extractorororororor0r0r0r (Autodesk Fusion 360 design; units mm, degrees)
Autodesk Fusion 360 part; units mm, degrees
sketch "Sketch1" plane through (0, 0, 0) normal (0, 1, 0) x (1, 0, 0)
  circle A0 centre (0, 0) radius 63.5
  line L0 (63.5, 63.5) -> (-63.5, 63.5)
  line L1 (-63.5, 63.5) -> (-63.5, -63.5)
  line L2 (-63.5, -63.5) -> (63.5, -63.5)
  line L3 (63.5, -63.5) -> (63.5, 63.5)
  line L4 (63.5, 63.5) -> (-63.5, -63.5) construction
  line L5 (-63.5, 63.5) -> (63.5, -63.5) construction
  line L6 (70, 70) -> (-70, 70)
  line L7 (-70, 70) -> (-70, -70)
  line L8 (-70, -70) -> (70, -70)
  line L9 (70, -70) -> (70, 70)
  line L10 (70, 70) -> (-70, -70) construction
  line L11 (-70, 70) -> (70, -70) construction
  circle A1 centre (0, 0) radius 70
  line L12 (60, 60) -> (-60, 60)
  line L13 (-60, 60) -> (-60, -60)
  line L14 (-60, -60) -> (60, -60)
  line L15 (60, -60) -> (60, 60)
  line L16 (60, 60) -> (-60, -60) construction
  line L17 (-60, 60) -> (60, -60) construction
  dimension "d1" = 127
  dimension "d2" = 127
  dimension "d3" = 127
  dimension "d4" = 140
  dimension "d5" = 140
  dimension "d14" = 120
  dimension "d15" = 120
  constraint coincident A0.centre A1.centre
  constraint perpendicular L0 L1
  constraint parallel L0 L2
  constraint parallel L1 L3
  constraint horizontal L0
  constraint coincident L4 A0.centre
  constraint coincident L5 A0.centre
  constraint perpendicular L6 L7
  constraint parallel L6 L8
  constraint parallel L7 L9
  constraint horizontal L6
  constraint coincident L10 A0.centre
  constraint coincident L11 A0.centre
  constraint tangent L8 A1
  constraint perpendicular L12 L13
  constraint parallel L12 L14
  constraint parallel L13 L15
  constraint horizontal L12
  constraint coincident L16 A0.centre
  constraint coincident L17 A0.centre
  measures "d1" diameter of A0
  measures "d2" distance of L1.end L2.end
  measures "d3" distance of L0.end L1.end
  measures "d4" distance of L7.end L8.end
  measures "d5" distance of L6.end L7.end
  measures "d14" distance of L12.end L13.end
  measures "d15" distance of L13.end L14.end
extrude "Extrude1" add sketch "Sketch1" along normal blind 30 contours A0 L3 A1 L15 | L3 A1 | A0 L3 A1 L15 | A0 A1 L12 L15 | A0 A1 L14 L15 | A0 L0 A1 L12 | A0 L2 A1 L14 | L0 A1 | A0 L0 A1 L12 | A0 A1 L12 L13 | A0 L2 A1 L14 | L2 A1 | A0 A1 L13 L14 | A0 L1 A1 L13 | A0 L1 A1 L13 | L1 A1 makes body 1
extrude "Extrude2" add sketch "Sketch1" against normal blind 30 separate body contours A0 L3 A1 L15 | A0 L3 A1 L15 | A0 A1 L12 L15 | A0 A1 L14 L15 | L2 L3 A1 L14 L15 | L0 L3 A1 L12 L15 | A0 L0 A1 L12 | A1 L12 L15 | A0 L2 A1 L14 | A1 L14 L15 | A0 L0 A1 L12 | A0 A1 L12 L13 | A0 L2 A1 L14 | A0 A1 L13 L14 | L0 L1 A1 L12 L13 | A0 L1 A1 L13 | A1 L12 L13 | L1 L2 A1 L13 L14 | A0 L1 A1 L13 | A1 L13 L14 makes body 2
extrude "Extrude3" add sketch "Sketch1" against normal blind 20 separate body contours L2 L3 L8 L9 A1 | L0 L3 L6 L9 A1 | L0 L1 L6 L7 A1 | L1 L2 L7 L8 A1 makes body 3
extrude "Extrude4" add sketch "Sketch1" against normal blind 20 contours L3 A1 | L0 A1 | L2 A1 | L1 A1 bodies 1 2 3
extrude "Extrude5" add sketch "Sketch1" against normal blind 30 contours A0 L15 | A0 L12 | A0 L14 | A0 L13 bodies 1
fillet "Fillet1" radius 5 4 edges at (63.5, -20, 0) (0, -20, -63.5) (0, -20, 63.5) (-63.5, -20, 0) on bodies 1
